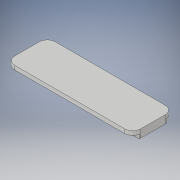
# Autodesk Inventor part: Cap
Saved by Autodesk Inventor 2019 (Build 230136000, 136)
## iProperties
Created: 2019-04-15
Part Number: Cap
Material: Generic
Document SubType Name: Modeling
Designer: Epsilon
Density: 1 g/cm^3
Appearance: Default
Author: Epsilon
Autodesk Inventor part; units mm, degrees
ref_plane "YZ Plane" through (0, 0, 0) normal (1, 0, 0) x (0, 1, 0)
ref_plane "XZ Plane" through (0, 0, 0) normal (0, 1, 0) x (-1, 0, 0)
ref_plane "XY Plane" through (0, 0, 0) normal (0, 0, 1) x (1, 0, 0)
sketch "Sketch1" plane through (0, 0, 0) normal (0, 1, 0) x (-1, 0, 0)
  line L0 (0, 0) -> (155, 0)
  line L1 (155, 0) -> (155, -50)
  line L2 (155, -50) -> (0, -50)
  line L3 (0, -50) -> (0, 0)
  dimension "d0" = 155
  dimension "d1" = 50
  constraints: 8 end point, 2 parallel, 1 horizontal, 1 perpendicular
  measures "d0" distance of L1.end L2.end
  measures "d1" distance between parallel lines of L2 L0
extrude "Extrusion1" add sketch "Sketch1" along normal blind 5
sketch "Sketch3" plane through (0, 0, 0) normal (0, -1, 0) x (1, 0, 0)
  line L0 (0, 0) -> (0, -50) projected
  line L1 (0, -42) -> (-70, -42)
  line L2 (-70, -42) -> (-70, -8)
  line L3 (-70, -8) -> (0, -8)
  line L4 (0, -8) -> (0, -42)
  line L5 (0, 0) -> (-155, 0) projected
  line L6 (-155, -50) -> (0, -50) projected
  line L7 (-78, -5.5) -> (-150, -5.5)
  line L8 (-150, -5.5) -> (-150, -44.5)
  line L9 (-150, -44.5) -> (-78, -44.5)
  line L10 (-78, -44.5) -> (-78, -5.5)
  dimension "d11" = 8
  dimension "d12" = 8
  dimension "d13" = 70
  dimension "d14" = 8
  dimension "d15" = 5.5
  dimension "d16" = 5.5
  dimension "d17" = 72
  constraints: 16 end point, 4 parallel, 2 horizontal, 2 perpendicular, 1 point on line
  measures "d11" distance between parallel lines of L5 L3
  measures "d12" distance between parallel lines of L6 L1
  measures "d13" distance between parallel lines of L2 L0
  measures "d14" distance between parallel lines of L10 L2
  measures "d15" distance between parallel lines of L6 L9
  measures "d16" distance between parallel lines of L5 L7
  measures "d17" distance between parallel lines of L8 L10
extrude "Extrusion3" add sketch "Sketch3" along normal blind 5
fillet "Fillet2" radius 10 4 edges at (0, 2.5, 0) (0, 2.5, -50) (-155, 2.5, 0) (-155, 2.5, -50)
equation "\"d12\" = d11"
equation "\"d16\" = d15"
body "Solid1"
